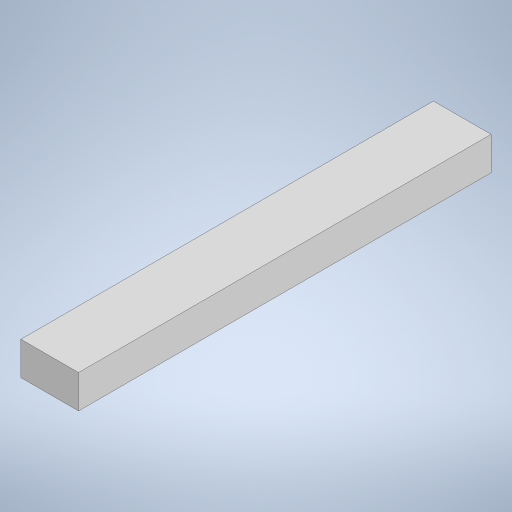
# Autodesk Inventor part: RectMiddleEyes
Saved by Autodesk Inventor 2024.3 (Build 283343000, 343)
## iProperties
Created: 2024-06-20
Part Number: RectMiddleEyes
Material: 一般
Document SubType Name: Modeling
Designer: yukin
Density: 1 g/cm^3
Appearance: 既定
Author: yukin
Autodesk Inventor part; units mm, degrees
ref_plane "YZ Plane" through (0, 0, 0) normal (1, 0, 0) x (0, 1, 0)
ref_plane "XZ Plane" through (0, 0, 0) normal (0, 1, 0) x (-1, 0, 0)
ref_plane "XY Plane" through (0, 0, 0) normal (0, 0, 1) x (1, 0, 0)
sketch "スケッチ1" plane through (0, 0, 0) normal (0, 1, 0) x (-1, 0, 0)
  line L0 (-16.777, 9.6054) -> (-19.377, 9.6054)
  line L1 (-19.377, 9.6054) -> (-19.377, -8.9946)
  line L2 (-19.377, -8.9946) -> (-16.777, -8.9946)
  line L3 (-16.777, -8.9946) -> (-16.777, 9.6054)
  point P0 (0, 0)
  dimension "d0" = 2.6
  dimension "d1" = 18.6
  constraints: 8 end point, 2 parallel, 1 horizontal, 1 perpendicular
  measures "d0" distance of L2.end L1.end
  measures "d1" distance of L1.end L0.end
extrude "押し出し1" add sketch "スケッチ1" along normal blind 1.5
